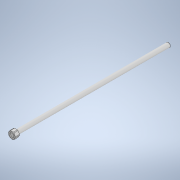
# Autodesk Inventor part: Through bolt
Saved by Autodesk Inventor 2022.4 (Build 264492000, 492)
## iProperties
Created: 2024-04-25
Part Number: Through bolt
Material: Generic
Document SubType Name: Modeling
Designer: t60147996
Density: 1 g/cm^3
Appearance: Default
Author: t60147996
Autodesk Inventor part; units mm, degrees
ref_plane "YZ Plane" through (0, 0, 0) normal (1, 0, 0) x (0, 1, 0)
ref_plane "XZ Plane" through (0, 0, 0) normal (0, 1, 0) x (-1, 0, 0)
ref_plane "XY Plane" through (0, 0, 0) normal (0, 0, 1) x (1, 0, 0)
sketch "Sketch2" plane through (0, 0, 0) normal (0, 0, 1) x (1, 0, 0)
  circle A0 centre (0, 0) radius 6.35
  dimension "d0" = 12.7
  constraints: 1 centre point, 1 coincident
  measures "d0" diameter of A0
extrude "Extrusion1" add sketch "Sketch2" along normal mid plane 441.96
chamfer "Chamfer1" distance 1.27 angle 45 1 edges at (-6.35, 0, -220.98)
sketch "Sketch3" plane through (0, 0, 220.98) normal (0, 0, 1) x (1, 0, 0)
  line L0 (10.9985, 0) -> (5.4993, -9.525)
  line L1 (5.4993, -9.525) -> (-5.4993, -9.525)
  line L2 (-5.4993, -9.525) -> (-10.9985, 0)
  line L3 (-10.9985, 0) -> (-5.4993, 9.525)
  line L4 (-5.4993, 9.525) -> (5.4993, 9.525)
  line L5 (5.4993, 9.525) -> (10.9985, 0)
  point P0 (0, 0)
  point P1 (0, 0)
  dimension "d6" = 19.05
  constraints: 12 end point, 1 coincident, 13 other
  measures "d6" distance between parallel lines of L1 L4
extrude "Extrusion2" add sketch "Sketch3" along normal blind 12.7
sketch "Sketch4" plane through (0, 0, 233.68) normal (0, 0, 1) x (1, 0, 0)
  circle A0 centre (0, 0) radius 6.35
  constraints: 1 centre point, 1 coincident
extrude "Extrusion3" cut sketch "Sketch4" against normal blind 2.54
sketch "Sketch5" plane through (0, 0, 0) normal (1, 0, 0) x (0, 1, 0)
  line L0 (0, 233.68) -> (9.525, 233.68) projected
  line L1 (9.525, 233.68) -> (11.1053, 233.68) construction
  line L2 (13.1997, 229.5016) -> (7.8979, 234.7834)
  line L3 (7.8979, 234.7834) -> (10.6425, 234.7834)
  line L4 (10.6425, 234.7834) -> (13.1997, 229.5016)
  line L5 (0, -312.1327) -> (0, 325.9361) projected
  point P0 (0, 0)
  constraints: 8 end point, 1 horizontal, 1 parallel
revolve "Revolution1" cut sketch "Sketch5" angle 360 about axis through (0, 0, -10) along (0, 0, 1)
chamfer "Chamfer2" distance 1.27 angle 45 6 edges at (5.4993, 9.525, 226.3372) (10.9985, 0, 226.3372) (5.4993, -9.525, 226.3372) (-5.4993, -9.525, 226.3372) (-10.9985, 0, 226.3372) (-5.4993, 9.525, 226.3372)
body "Solid1"
